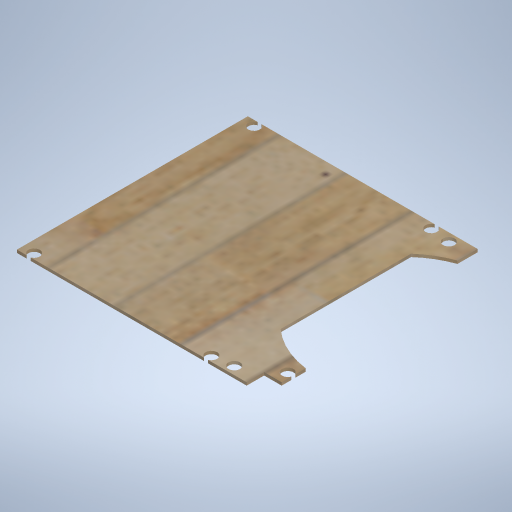
# Autodesk Inventor part: base
Saved by Autodesk Inventor 2024.1 (Build 281209000, 209)
## iProperties
Created: 2025-09-27
Part Number: base
Material: 木材 (カエデ材)
Document SubType Name: Modeling
Designer: hibik
Density: 0.67 g/cm^3
Appearance: ナチュラル カエデ材 - 光沢 濃い着色
Author: hibik
Autodesk Inventor part; units mm, degrees
ref_plane "YZ Plane" through (0, 0, 0) normal (1, 0, 0) x (0, 1, 0)
ref_plane "XZ Plane" through (0, 0, 0) normal (0, 1, 0) x (-1, 0, 0)
ref_plane "XY Plane" through (0, 0, 0) normal (0, 0, 1) x (1, 0, 0)
sketch "スケッチ1" plane through (0, 0, 0) normal (0, 1, 0) x (-1, 0, 0)
  line L0 (0, 99) -> (172, 99)
  line L1 (172, 99) -> (172, -99)
  line L2 (172, -99) -> (0, -99)
  line L3 (0, -99) -> (0, 99)
  line L4 (20, 99) -> (20, -99)
  line L5 (142, 99) -> (142, -99)
  point P0 (0, 0)
  point P1 (0, 0)
  dimension "d0" = 198
  dimension "d3" = 20
  dimension "d4" = 122
  dimension "d5" = 30
  constraints: 12 end point, 4 point on line, 2 parallel, 2 perpendicular, 1 coincident, 1 horizontal, 1 midpoint, 1 vertical
  measures "d0" distance of L0.end L1.end
  measures "d3" distance between parallel lines of L3 L4
  measures "d4" distance between parallel lines of L4 L5
  measures "d5" distance between parallel lines of L5 L1
extrude "押し出し1" add sketch "スケッチ1" along normal blind 2.5
sketch "スケッチ3" plane through (0, 2.5, 0) normal (0, 1, 0) x (1, 0, 0)
  line L0 (25, -99) -> (0, -99)
  line L1 (0, -99) -> (0, -84)
  line L2 (0, -84) -> (25, -84)
  line L3 (25, -84) -> (25, -99)
  line L4 (0, -99) -> (0, 99) projected
  line L5 (-172, -99) -> (0, -99) projected
  line L6 (0, -84) -> (40, -84)
  line L7 (40, -84) -> (40, -64)
  line L8 (40, -64) -> (0, -64)
  line L9 (0, -64) -> (0, -84)
  line L10 (-20, 99) -> (-20, -99) projected
  circle A0 centre (50, 11) radius 70
  circle A1 centre (50, 11) radius 75
  line L11 (0, 99) -> (25, 99)
  line L12 (25, 99) -> (25, 84)
  line L13 (25, 84) -> (0, 84)
  line L14 (0, 84) -> (0, 99)
  line L15 (25, 84) -> (25, 81.7107)
  line L16 (40, -64) -> (40, -63.3303)
  point P0 (0, 0)
  point P1 (0, -64)
  point P2 (0, 66.9017)
  point P3 (0, -44.9017)
  dimension "d16" = 15
  dimension "d17" = 40
  dimension "d18" = 20
  dimension "d19" = 25
  dimension "d23" = 140
  dimension "d24" = 5
  dimension "d25" = 110
  dimension "d26" = 60
  constraints: 28 end point, 8 parallel, 3 horizontal, 3 perpendicular, 2 centre point, 2 collinear, 2 equal length, 2 point on circle, 2 tangent, 1 coincident
  measures "d16" distance of L2.end L0.start
  measures "d17" distance of L7.end L8.end
  measures "d18" distance of L6.end L7.end
  measures "d19" distance of L0.start L0.end
  measures "d23" diameter of A0
  measures "d24" radial gap between concentric circles of A1 A0
  measures "d25" distance from line of L5 A0.centre
  measures "d26" distance between parallel lines of L10 L7
extrude "押し出し4" add sketch "スケッチ3" against normal up to surface (2.5 mm away) contours L0 L1 L2 L3 | L2 L4 L8 L7 L6 | L4 A1 L16 L8 | L4 L13 L15 A1 | L4 L11 L12 L13
sketch "スケッチ4" plane through (0, 2.5, 0) normal (0, 1, 0) x (1, 0, 0)
  circle A0 centre (-10, -94.3) radius 1.6 projected
  circle A1 centre (-10, 94.3) radius 1.6 projected
  circle A2 centre (7.35, 92) radius 1.6 projected
  line L0 (5, -90.6432) -> (7.35, -89.2865) projected
  circle A3 centre (7.35, -92) radius 1.6 projected
  circle A4 centre (35.3, -74) radius 1.6 projected
  circle A5 centre (-162, -94.3) radius 1.6 projected
  circle A6 centre (-162, 94.3) radius 1.6 projected
  circle A7 centre (-162, -94.3) radius 5
  circle A8 centre (-162, 94.3) radius 5
  circle A9 centre (-10, -94.3) radius 5
  circle A10 centre (-10, 94.3) radius 5
  circle A11 centre (7.35, 92) radius 5
  circle A12 centre (7.35, -92) radius 5
  circle A13 centre (35.3, -74) radius 5
  point P0 (0, 0)
  dimension "d27" = 10
  constraints: 7 centre point, 7 coincident, 6 equal radius
  measures "d27" diameter of A7
extrude "押し出し5" cut sketch "スケッチ4" against normal through all contours A0 | A1 | A2 | A3 | A4 | A5 | A6 | A7 | A8 | A9 | A10 | A11 | A12 | A13
